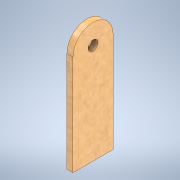
# Autodesk Inventor part: Conveyor Stand
Saved by Autodesk Inventor 2022.2 (Build 262287000, 287)
## iProperties
Created: 2022-02-27
Part Number: Conveyor Stand
Material: Pine, Southern
Document SubType Name: Modeling
Designer: PRASHANTH
Density: 0.570257 g/cm^3
Appearance: Yellow Pine - Stained Dark Medium Gloss
Author: PRASHANTH
Autodesk Inventor part; units mm, degrees
ref_plane "YZ Plane" through (0, 0, 0) normal (1, 0, 0) x (0, 1, 0)
ref_plane "XZ Plane" through (0, 0, 0) normal (0, 1, 0) x (-1, 0, 0)
ref_plane "XY Plane" through (0, 0, 0) normal (0, 0, 1) x (1, 0, 0)
sketch "Sketch1" plane through (0, 0, 0) normal (1, 0, 0) x (0, 1, 0)
  line L0 (20, 10) -> (-30, 10)
  line L1 (-30, 10) -> (-30, -10)
  line L2 (-30, -10) -> (20, -10)
  arc A0 (20, -10) -> (20, 10) centre (20, 0) ccw
  circle A1 centre (20, 0) radius 2.5
  point P0 (0, 0)
  constraints: 6 end point, 2 centre point, 2 point on circle, 2 tangent, 1 coincident, 1 horizontal, 1 parallel, 1 perpendicular
extrude "Extrusion1" add sketch "Sketch1" along normal blind 3
body "Solid1"
